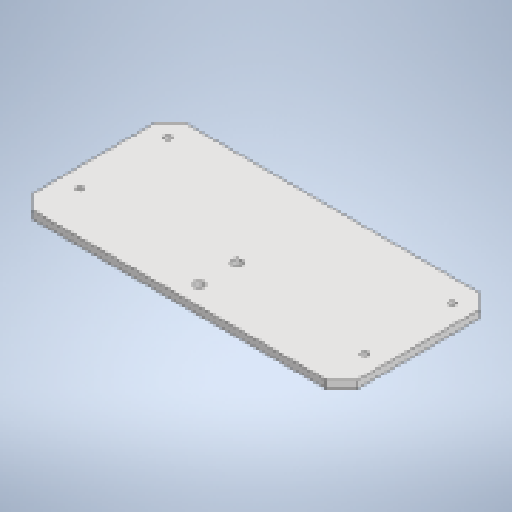
# Autodesk Inventor part: фанера
Saved by Autodesk Inventor 2023.1 (Build 271208000, 208)
## iProperties
Created: 2025-12-23
Part Number: фанера
Material: Типовые
Document SubType Name: Modeling
Designer: DELL
Density: 1 g/cm^3
Appearance: По умолчанию
Author: DELL
Autodesk Inventor part; units mm, degrees
ref_plane "YZ Plane" through (0, 0, 0) normal (1, 0, 0) x (0, 1, 0)
ref_plane "XZ Plane" through (0, 0, 0) normal (0, 1, 0) x (-1, 0, 0)
ref_plane "XY Plane" through (0, 0, 0) normal (0, 0, 1) x (1, 0, 0)
sketch "Эскиз1" plane through (0, 0, 0) normal (0, 1, 0) x (-1, 0, 0)
  line L0 (85.25, 40) -> (-85.25, 40)
  line L1 (-85.25, 40) -> (-85.25, -40)
  line L2 (-85.25, -40) -> (85.25, -40)
  line L3 (85.25, -40) -> (85.25, 40)
  line L4 (85.25, 40) -> (-85.25, -40) construction
  line L5 (-85.25, 40) -> (85.25, -40) construction
  point P0 (0, 0)
  dimension "d0" = 170.5
  dimension "d1" = 80
  constraints: 12 end point, 2 midpoint, 2 parallel, 1 horizontal, 1 perpendicular
  measures "d0" distance of L2.end L1.end
  measures "d1" distance of L1.end L0.end
extrude "Выдавливание1" add sketch "Эскиз1" along normal blind 4
sketch "Эскиз2" plane through (0, 4, 0) normal (0, 1, 0) x (1, 0, 0)
  circle A0 centre (75.25, -18) radius 1.6 projected
  circle A1 centre (-75.25, 28.7) radius 1.6 projected
  circle A2 centre (75.25, 28.2) radius 1.6 projected
  circle A3 centre (-75.25, -17.5) radius 1.6 projected
  point P0 (0, 0)
extrude "Выдавливание2" cut sketch "Эскиз2" against normal blind 4
chamfer "Фаска1" distance 8 angle 45 4 edges at (-85.25, 2, -40) (-85.25, 2, 40) (85.25, 2, -40) (85.25, 2, 40)
sketch "Эскиз3" plane through (0, 4, 0) normal (0, 1, 0) x (1, 0, 0)
  circle A0 centre (0, -30) radius 2.55
  circle A1 centre (0, -10) radius 2.55
  line L0 (-85.25, 32) -> (-85.25, -32) projected
  line L1 (-77.25, -40) -> (77.25, -40) projected
  point P0 (0, 0)
  dimension "d11" = 85.25
  dimension "d12" = 10
  dimension "d13" = 5.1
  constraints: 2 centre point
  measures "d11" distance from line of L0 A0.centre
  measures "d12" distance from line of L1 A0.centre
  measures "d13" diameter of A0
extrude "Выдавливание3" cut sketch "Эскиз3" against normal blind 10
